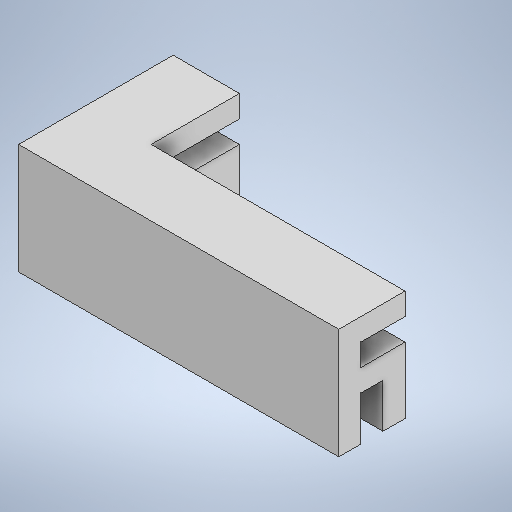
# Autodesk Inventor part: TSU_Corner2_Clamp
Saved by Autodesk Inventor 2025.2 (Build 292293000, 293)
## iProperties
Created: 2025-01-07
Part Number: TSU_Corner2_Clamp
Material: Generic
Document SubType Name: Modeling
Designer: Matt Tidd
Density: 1 g/cm^3
Appearance: Default
Author: Matt Tidd
Autodesk Inventor part; units mm, degrees
ref_plane "YZ Plane" through (0, 0, 0) normal (1, 0, 0) x (0, 1, 0)
ref_plane "XZ Plane" through (0, 0, 0) normal (0, 1, 0) x (-1, 0, 0)
ref_plane "XY Plane" through (0, 0, 0) normal (0, 0, 1) x (1, 0, 0)
sketch "Sketch1" plane through (0, 0, 0) normal (0, 1, 0) x (-1, 0, 0)
  line L0 (0, 0) -> (145, 0)
  line L1 (145, 0) -> (145, -30)
  line L2 (145, -30) -> (0, -30)
  line L3 (0, -30) -> (0, 0)
  line L4 (145, 0) -> (115, 0)
  line L5 (115, 0) -> (115, -70)
  line L6 (115, -70) -> (145, -70)
  line L7 (145, -70) -> (145, 0)
  point P0 (115, -30)
  dimension "d0" = 145
  dimension "d1" = 30
  dimension "d2" = 30
  dimension "d3" = 70
  constraints: 16 end point, 4 parallel, 2 horizontal, 2 perpendicular
  measures "d0" distance of L1.end L2.end
  measures "d1" distance of L0.end L1.end
  measures "d2" distance of L6.end L5.end
  measures "d3" distance of L5.end L4.end
extrude "Extrusion1" add sketch "Sketch1" along normal blind 30
sketch "Sketch2" plane through (0, 0, -30) normal (0, 0, -1) x (-1, 0, 0)
  line L0 (0, 0) -> (0, 30) projected
  line L1 (0, 20) -> (135, 20)
  line L2 (135, 20) -> (135, 10)
  line L3 (135, 10) -> (0, 10)
  line L4 (0, 10) -> (0, 20)
  point P0 (0, 10)
  dimension "d26" = 135
  dimension "d27" = 10
  constraints: 8 end point, 2 parallel, 1 horizontal, 1 perpendicular, 1 point on line
  measures "d26" distance of L2.end L3.end
  measures "d27" distance of L1.end L2.end
extrude "Extrusion2" cut sketch "Sketch2" along normal blind 50 and the other way blind 20
sketch "Sketch5" plane through (0, 0, 0) normal (0, -1, 0) x (1, 0, 0)
  line L0 (-145, -70) -> (-145, 0) projected
  line L1 (-145, 0) -> (0, 0)
  line L2 (0, 0) -> (0, -10)
  line L3 (0, -10) -> (-145, -10)
  line L4 (-145, -10) -> (-145, 0)
  line L5 (-115, -70) -> (-145, -70) projected
  line L6 (-145, -10) -> (-135, -10)
  line L7 (-135, -10) -> (-135, -70)
  line L8 (-135, -70) -> (-145, -70)
  line L9 (-145, -70) -> (-145, -10)
  line L10 (-115, -70) -> (-125, -70)
  line L11 (-125, -70) -> (-125, -30)
  line L12 (-125, -30) -> (-115, -30)
  line L13 (-115, -30) -> (-115, -70)
  line L14 (-125, -30) -> (0, -30)
  line L15 (0, -30) -> (0, -20)
  line L16 (0, -20) -> (-125, -20)
  line L17 (-125, -20) -> (-125, -30)
  point P0 (0, 0)
  dimension "d28" = 145
  dimension "d29" = 10
  dimension "d30" = 10
  dimension "d31" = 10
  dimension "d32" = 10
  constraints: 32 end point, 8 parallel, 4 horizontal, 4 perpendicular, 3 point on line
  measures "d28" distance of L2.end L3.end
  measures "d29" distance of L1.end L2.end
  measures "d30" distance of L7.end L8.end
  measures "d31" distance of L11.end L12.end
  measures "d32" distance of L15.end L14.end
extrude "Extrusion5" add sketch "Sketch5" along normal blind 20
body "Solid1"
